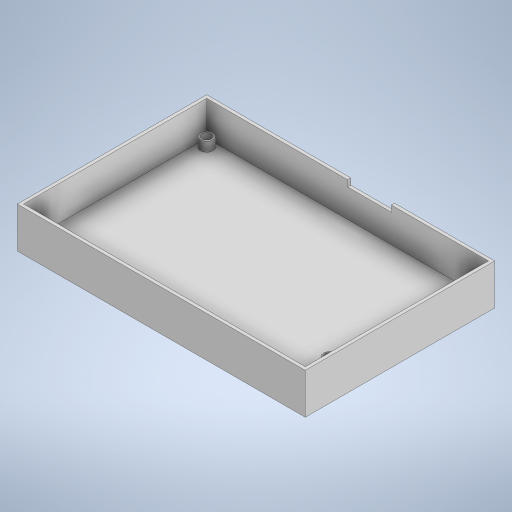
# Autodesk Inventor part: base_traseira
Saved by Autodesk Inventor 2023 (Build 270158000, 158)
## iProperties
Created: 2022-11-25
Part Number: base_traseira
Material: Genérico
Document SubType Name: Modeling
Designer: Inteli
Density: 1 g/cm^3
Appearance: Padrão
Author: Inteli
## iProperties of the stored document base_traseira_3DPrint.ipt
Created: 2022-11-29
Part Number: base_traseira_3DPrint
Material: Genérico
Document SubType Name: Modeling
Designer: Inteli
Density: 1 g/cm^3
Appearance: Padrão
Author: Inteli
Autodesk Inventor part; units mm, degrees
ref_plane "YZ Plane" through (0, 0, 0) normal (1, 0, 0) x (0, 1, 0)
ref_plane "XZ Plane" through (0, 0, 0) normal (0, 1, 0) x (-1, 0, 0)
ref_plane "XY Plane" through (0, 0, 0) normal (0, 0, 1) x (1, 0, 0)
sketch "Base" plane through (0, 0, 0) normal (0, 1, 0) x (-1, 0, 0)
  line L0 (92, 60.5) -> (-92, 60.5)
  line L1 (-92, 60.5) -> (-92, -60.5)
  line L2 (-92, -60.5) -> (92, -60.5)
  line L3 (92, -60.5) -> (92, 60.5)
  line L4 (92, 60.5) -> (-92, -60.5) construction
  line L5 (-92, 60.5) -> (92, -60.5) construction
  point P0 (0, 0)
  dimension "d0" = 184
  dimension "d1" = 121
  constraints: 12 end point, 2 midpoint, 2 parallel, 1 horizontal, 1 perpendicular
  measures "d0" distance of L2.end L1.end
  measures "d1" distance of L1.end L0.end
extrude "Extrusão1" add sketch "Base" against normal blind 26
sketch "Esboço2" plane through (0, 0, 0) normal (0, 1, 0) x (1, 0, 0)
  line L0 (-90, -58.5) -> (90, -58.5)
  line L1 (90, -58.5) -> (90, 58.5)
  line L2 (90, 58.5) -> (-90, 58.5)
  line L3 (-90, 58.5) -> (-90, -58.5)
  line L4 (-90, -58.5) -> (90, 58.5) construction
  line L5 (90, -58.5) -> (-90, 58.5) construction
  point P0 (0, 0)
  dimension "d4" = 180
  dimension "d5" = 117
  constraints: 12 end point, 2 midpoint, 2 parallel, 1 horizontal, 1 perpendicular
  measures "d4" distance of L2.end L1.end
  measures "d5" distance of L1.end L0.end
extrude "Extrusão2" cut sketch "Esboço2" against normal blind 22
sketch "Esboço3" plane through (0, -22, 0) normal (0, 1, 0) x (1, 0, 0)
  circle A0 centre (-85, -53.5) radius 4
  line L0 (-92, 60.5) -> (-92, -60.5) projected
  line L1 (-92, -60.5) -> (92, -60.5) projected
  circle A1 centre (-85, -53.5) radius 3
  line L2 (-90, -58.5) -> (-90, 58.5) projected
  line L3 (90, 58.5) -> (90, -58.5) projected
  circle A2 centre (-85, 53.5) radius 4
  circle A3 centre (-85, 53.5) radius 3
  line L4 (-90, 58.5) -> (90, 58.5) projected
  line L5 (90, -58.5) -> (-90, -58.5) projected
  circle A4 centre (85, 53.5) radius 3
  circle A5 centre (85, 53.5) radius 4
  line L6 (92, -60.5) -> (92, 60.5) projected
  line L7 (92, 60.5) -> (-92, 60.5) projected
  circle A6 centre (76.27, -28.99) radius 4
  circle A7 centre (76.27, -28.99) radius 3
  point P0 (0, 0)
  dimension "d8" = 8
  dimension "d9" = 7
  dimension "d10" = 7
  dimension "d11" = 6
  dimension "d12" = 7
  dimension "d13" = 7
  dimension "d14" = 8
  dimension "d15" = 31.51
  dimension "d16" = 15.73
  dimension "d17" = 6
  dimension "d29" = 6
  dimension "d30" = 8
  dimension "d31" = 8
  dimension "d32" = 6
  constraints: 8 centre point, 4 coincident
  measures "d8" diameter of A0
  measures "d9" distance from line of L0 A0.centre
  measures "d10" distance from line of L1 A0.centre
  measures "d11" diameter of A1
  measures "d12" distance from line of L6 A4.centre
  measures "d13" distance from line of L7 A4.centre
  measures "d14" diameter of A6
  measures "d15" distance from line of L1 A6.centre
  measures "d16" distance from line of L6 A6.centre
  measures "d17" diameter of A7
  measures "d29" diameter of A3
  measures "d30" diameter of A2
  measures "d31" diameter of A5
  measures "d32" diameter of A4
extrude "Extrusão3" add sketch "Esboço3" along normal blind 6 contours A0 | A2 | A5 | A6
sketch "Esboço4" plane through (92, 0, -60.5) normal (0, 0, -1) x (-1, 0, 0)
  line L0 (92, 0) -> (64, 0)
  line L1 (64, 0) -> (64, -4)
  line L2 (64, -4) -> (92, -4)
  line L3 (92, -4) -> (92, 0)
  line L4 (92, 0) -> (64, -4) construction
  line L5 (64, 0) -> (92, -4) construction
  line L6 (184, 0) -> (184, -26) projected
  line L7 (0, 0) -> (184, 0) projected
  line L8 (184, -26) -> (0, -26) projected
  point P0 (92, 0)
  point P1 (78, -2)
  point P2 (64, -2)
  dimension "d20" = 120
  dimension "d21" = 28
  dimension "d22" = 0
  dimension "d24" = 4
  constraints: 12 end point, 3 midpoint, 2 parallel, 1 horizontal, 1 perpendicular
  measures "d20" distance between parallel lines of L1 L6
  measures "d21" distance from line of point (64, -2) L3
  measures "d22" distance between parallel lines of L7 L0
  measures "d24" distance of L2.end L0.start
extrude "Extrusão4" cut sketch "Esboço4" along normal blind 4 and the other way blind 2
